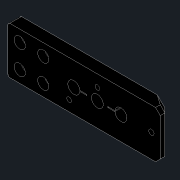
# Autodesk Inventor part: z-plate-bottom
Saved by Autodesk Inventor 2021 (Build 250183000, 183)
## iProperties
Company: Prusa Development a.s.
Created: 2019-03-18
Material: Všeobecné
Document SubType Name: Modeling
Density: 1 g/cm^3
Appearance: Hliník – tmavý
Project: ORIGINAL PRUSA MINI
Authority: Ing. Robert Turinský
Part Number: z-plate-bottom
Author: Ing. Robert Turinský
Title: MINI-z-plate-bottom
Revision Number: R4
## iProperties of the stored document _3DPrint.ipt
Created: 2021-05-23
Part Number: _3DPrint
Material: Generic
Document SubType Name: Modeling
Designer: arbra
Density: 1 g/cm^3
Appearance: Default
Author: arbra
Autodesk Inventor part; units mm, degrees
ref_plane "YZ Plane" through (0, 0, 0) normal (1, 0, 0) x (0, 1, 0)
ref_plane "XZ Plane" through (0, 0, 0) normal (0, 1, 0) x (-1, 0, 0)
ref_plane "XY Plane" through (0, 0, 0) normal (0, 0, 1) x (1, 0, 0)
sketch "Sketch1" plane through (0, 0, 0) normal (0, 0, 1) x (1, 0, 0)
  line L0 (49.5, 20) -> (-74.5, 20)
  line L1 (-76, 18.5) -> (-76, -18.5)
  line L2 (-74.5, -20) -> (49.5, -20)
  line L3 (-102.2728, 0) -> (79.4621, 0) construction
  line L4 (0, 28.4349) -> (0, -28.4349) construction
  circle A0 centre (0, 0) radius 5
  circle A1 centre (20, 0) radius 5.075
  line L5 (14.9389, 0.375) -> (8.9389, 0.375)
  line L6 (8.9389, 0.375) -> (8.9389, 0)
  line L7 (14.9389, -0.375) -> (8.9389, -0.375)
  line L8 (8.9389, -0.375) -> (8.9389, 0)
  circle A2 centre (-20, 0) radius 5.075
  line L9 (-14.9389, 0.375) -> (-8.9389, 0.375)
  line L10 (-8.9389, 0.375) -> (-8.9389, 0)
  line L11 (-14.9389, -0.375) -> (-8.9389, -0.375)
  line L12 (-8.9389, -0.375) -> (-8.9389, 0)
  circle A3 centre (0, 10) radius 2
  line L13 (36, 20) -> (36, -20) construction
  circle A4 centre (-24, -11) radius 2
  circle A5 centre (46, 0) radius 2.25
  line L14 (-46, -10) -> (-66, -10) construction
  line L15 (-66, -10) -> (-66, 10) construction
  line L16 (-66, 10) -> (-46, 10) construction
  line L17 (-46, 10) -> (-46, -10) construction
  line L18 (-46, -10) -> (-66, 10) construction
  line L19 (-66, -10) -> (-46, 10) construction
  circle A6 centre (-66, 10) radius 2.75
  circle A7 centre (-46, 10) radius 2.75
  circle A8 centre (-46, -10) radius 2.75
  circle A9 centre (-66, -10) radius 2.75
  line L20 (0, 15) -> (-45, 15) construction
  line L21 (-45, 15) -> (-45, 0) construction
  line L22 (-45, 0) -> (-30, -15) construction
  line L23 (-30, -15) -> (0, -15) construction
  line L24 (-36, -20) -> (-76, -20) construction
  line L25 (-76, -20) -> (-76, 20) construction
  line L26 (-76, 20) -> (-36, 20) construction
  line L27 (-36, 20) -> (-36, -20) construction
  line L28 (-36, -20) -> (-76, 20) construction
  line L29 (-76, -20) -> (-36, 20) construction
  arc A10 (-76, -18.5) -> (-74.5, -20) centre (-74.5, -18.5) ccw
  arc A11 (-74.5, 20) -> (-76, 18.5) centre (-74.5, 18.5) ccw
  line L30 (53.5, -16) -> (53.5, 16)
  line L31 (53.5, -16) -> (49.5, -20)
  line L32 (49.5, 20) -> (53.5, 16)
  point P0 (0, 0)
  point P1 (-56, 0)
  point P2 (53.5, -20)
  point P3 (53.5, 20)
  point P4 (-14.9389, -0.375)
  point P5 (14.9389, -0.375)
  dimension "d99" = 10.15
  dimension "d44" = 10
  dimension "d46" = 0.75
  dimension "d47" = 6
  dimension "d48" = 40
  dimension "d49" = 4
  dimension "d50" = 10
  dimension "d51" = 16
  dimension "d55" = 11
  dimension "d56" = 4
  dimension "d60" = 10
  dimension "d62" = 20
  dimension "d63" = 10
  dimension "d64" = 5.5
  dimension "d65" = 45
  dimension "d66" = 30
  dimension "d67" = 45
  dimension "d68" = 40
  dimension "d69" = 40
  dimension "d70" = 1.5
  dimension "d73" = 16
  dimension "d86" = 17.5
  dimension "d87" = 40
  dimension "d89" = 4.5
  dimension "d90" = 4
  dimension "d91" = 4
  dimension "d92" = 4
  dimension "d93" = 4
  constraints: 62 end point, 10 centre point, 9 point on line, 7 parallel, 7 perpendicular, 6 midpoint, 6 symmetric about line, 5 coincident, 5 equal radius, 5 horizontal, 4 point on circle, 4 tangent, 3 vertical, 2 vertical alignment, 14 other
  measures "d44" diameter of A0
  measures "d46" distance between parallel lines of L7 L5
  measures "d47" distance of L7.start L7.end
  measures "d48" distance of point (-20, 0) point (20, 0)
  measures "d49" diameter of A3
  measures "d50" distance of A3.centre A0.centre
  measures "d51" distance from line of point (20, 0) L13
  measures "d56" horizontal distance of A4.centre point (-20, 0)
  measures "d60" distance from line of L13 A5.centre
  measures "d62" distance of L15.end L16.end
  measures "d63" distance between parallel lines of L1 L15
  measures "d64" diameter of A6
  measures "d65" angle of L21 L22
  measures "d66" distance between parallel lines of L23 L20
  measures "d67" distance between parallel lines of L21 L4
  measures "d68" distance of L24.end L25.end
  measures "d69" distance between parallel lines of L27 L25
  measures "d70" radius of A10
  measures "d73" distance from line of L27 point (-20, 0)
  measures "d86" distance between parallel lines of L30 L13
  measures "d87" distance between parallel lines of L0 L2
  measures "d89" diameter of A5
  measures "d90" distance of L30.start point (53.5, -20)
  measures "d91" distance of L2.end point (53.5, -20)
  measures "d92" distance of L0.start point (53.5, 20)
  measures "d93" distance of L30.end point (53.5, 20)
extrude "Vysunutí1" add sketch "Sketch1" along normal blind 10
sketch "Sketch2" plane through (0, 0, 0) normal (0, 0, -1) x (-1, 0, 0)
  circle A0 centre (-46, 0) radius 2.25 construction
  circle A1 centre (-46, 0) radius 2.25 projected
  circle A2 centre (-46, 0) radius 4
  circle A3 centre (0, 10) radius 2 construction
  circle A4 centre (24, -11) radius 2 construction
  circle A5 centre (0, 10) radius 3
  circle A6 centre (24, -11) radius 3
  point P0 (0, 0)
  point P1 (-66, 0)
  dimension "d85" = 6
  constraints: 3 centre point, 3 coincident, 1 equal radius
  measures "d85" diameter of A5
extrude "Extrusion2" cut sketch "Sketch2" against normal blind 5 contours A1 | A2 | A5 | A6
sketch "Sketch3" plane through (0, 0, 10) normal (0, 0, 1) x (1, 0, 0)
  circle A0 centre (-46, -10) radius 2.75 construction
  circle A1 centre (-66, -10) radius 2.75 construction
  circle A2 centre (-66, 10) radius 2.75 construction
  circle A3 centre (-46, 10) radius 2.75 construction
  circle A4 centre (-46, -10) radius 2.75 construction
  circle A5 centre (-46, -10) radius 4.75
  circle A6 centre (-66, -10) radius 4.75
  circle A7 centre (-66, 10) radius 4.75
  circle A8 centre (-46, 10) radius 4.75
  point P0 (0, 0)
  dimension "d82" = 9.5
  constraints: 4 centre point, 4 coincident, 3 equal radius
  measures "d82" diameter of A5
extrude "Extrusion3" cut sketch "Sketch3" against normal blind 6
chamfer "Chamfer1" distance 6 angle 45 3 edges at (53.5, 0, 0) (51.5, -18, 0) (51.5, 18, 0)
